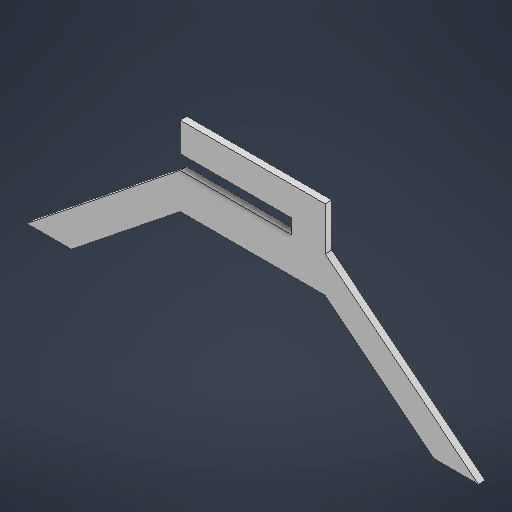
# Autodesk Inventor part: Support_base
Saved by Autodesk Inventor 2027 (Build 310192000, 192)
## iProperties
Created: 2026-05-13
Part Number: Support_base
Material: Generic
Document SubType Name: Modeling
Designer: alexy
Density: 1 g/cm^3
Appearance: Default
Author: alexy
Autodesk Inventor part; units mm, degrees
ref_plane "YZ Plane" through (0, 0, 0) normal (1, 0, 0) x (0, 1, 0)
ref_plane "XZ Plane" through (0, 0, 0) normal (0, 1, 0) x (-1, 0, 0)
ref_plane "XY Plane" through (0, 0, 0) normal (0, 0, 1) x (1, 0, 0)
sketch "Sketch1" plane through (0, 0, 0) normal (0, 0, 1) x (1, 0, 0)
  line L0 (0, 19.5) -> (50, 19.5)
  line L1 (50, 19.5) -> (50, 6.5)
  line L2 (50, 6.5) -> (0, 6.5)
  line L3 (0, 6.5) -> (0, 19.5)
  line L4 (50, 19.5) -> (65, 19.5)
  line L5 (65, 19.5) -> (65, 0)
  line L6 (65, 0) -> (50, 0)
  line L7 (50, 0) -> (50, 19.5)
  line L8 (65, 0) -> (0, 0)
  line L9 (0, 0) -> (0, -16)
  line L10 (0, -16) -> (65, -16)
  line L11 (65, -16) -> (65, 0)
  line L12 (0, 0) -> (-68.75, -55)
  line L13 (-68.75, -55) -> (-48.75, -55)
  line L14 (-48.75, -55) -> (0, -16)
  line L15 (65, -16) -> (113.75, -55)
  line L16 (113.75, -55) -> (133.75, -55)
  line L17 (133.75, -55) -> (65, 0)
  point P0 (50, 6.5)
  point P1 (50, 0)
  dimension "d0" = 6.5
  dimension "d1" = 13
  dimension "d2" = 50
  dimension "d3" = 15
  dimension "d4" = 16
  dimension "d5" = 20
  dimension "d6" = 20
  dimension "d7" = 55
  constraints: 36 end point, 8 parallel, 4 horizontal, 3 perpendicular, 2 point on line, 1 coincident, 1 horizontal alignment, 1 vertical alignment
  measures "d0" distance from line of point (0, 0) L2
  measures "d1" distance of L2.end L0.start
  measures "d2" distance of L0.start L0.end
  measures "d3" distance of L0.end L4.end
  measures "d4" distance of L8.end L9.end
  measures "d5" distance of L12.end L13.end
  measures "d6" distance of L15.end L16.end
  measures "d7" vertical distance of L16.end L5.end
extrude "Extrusion1" add sketch "Sketch1" along normal blind 3
body "Solid1"
